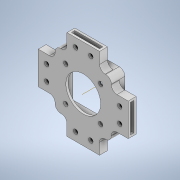
# Autodesk Inventor part: CSB_Motor_Mount_v1
Saved by Autodesk Inventor 2021 (Build 250183000, 183)
## iProperties
Created: 2023-12-30
Part Number: CSB_Motor_Mount_v1
Material: Generic
Document SubType Name: Modeling
Designer: brybr
Density: 1 g/cm^3
Appearance: Default
Author: brybr
Autodesk Inventor part; units mm, degrees
ref_plane "YZ Plane" through (0, 0, 0) normal (1, 0, 0) x (0, 1, 0)
ref_plane "XZ Plane" through (0, 0, 0) normal (0, 1, 0) x (-1, 0, 0)
ref_plane "XY Plane" through (0, 0, 0) normal (0, 0, 1) x (1, 0, 0)
sketch "Sketch1" plane through (0, 0, 0) normal (0, 0, 1) x (1, 0, 0)
  line L0 (-15.5, 15.5) -> (15.5, 15.5) construction
  line L1 (15.5, 15.5) -> (15.5, -15.5) construction
  line L2 (15.5, -15.5) -> (-15.5, -15.5) construction
  line L3 (-15.5, -15.5) -> (-15.5, 15.5) construction
  line L4 (-15.5, 15.5) -> (15.5, -15.5) construction
  line L5 (15.5, 15.5) -> (-15.5, -15.5) construction
  circle A0 centre (-15.5, 15.5) radius 2
  circle A1 centre (15.5, 15.5) radius 2
  circle A2 centre (-15.5, -15.5) radius 2
  circle A3 centre (15.5, -15.5) radius 2
  line L6 (-21.25, 21.25) -> (21.25, 21.25)
  line L7 (21.25, 21.25) -> (21.25, -21.25)
  line L8 (21.25, -21.25) -> (-21.25, -21.25)
  line L9 (-21.25, -21.25) -> (-21.25, 21.25)
  line L10 (-21.25, 21.25) -> (21.25, -21.25) construction
  line L11 (21.25, 21.25) -> (-21.25, -21.25) construction
  circle A4 centre (0, 0) radius 15.5
  line L12 (25, -25) -> (-25, -25)
  line L13 (-25, -25) -> (-25, 25)
  line L14 (-25, 25) -> (25, 25)
  line L15 (25, 25) -> (25, -25)
  line L16 (25, -25) -> (-25, 25) construction
  line L17 (-25, -25) -> (25, 25) construction
  dimension "d0" = 31
  dimension "d1" = 31
  dimension "d2" = 4
  dimension "d5" = 31
  dimension "d8" = 31
  dimension "d11" = 42.5
  dimension "d12" = 42.5
  dimension "d13" = 50
  dimension "d14" = 50
  constraints: 36 end point, 6 midpoint, 6 parallel, 5 centre point, 4 horizontal, 3 perpendicular, 2 coincident, 1 vertical, 6 other
  measures "d0" distance of L1.end L2.end
  measures "d1" distance of L0.end L1.end
  measures "d2" diameter of A0
  measures "d5" distance of A0.centre A1.centre
  measures "d8" distance of A0.centre A2.centre
  measures "d11" distance of L7.end L8.end
  measures "d12" distance of L6.end L7.end
  measures "d13" distance of L13.end L14.end
  measures "d14" distance of L12.end L13.end
extrude "Extrusion1" add sketch "Sketch1" along normal blind 2 contours L6 L7 L8 L9 | L12 L13 L14 L15
extrude "Extrusion2" add sketch "Sketch1" against normal blind 10 contours L12 L13 L14 L15
sketch "Sketch2" plane through (-25, -25, 2) normal (-1, 0, 0) x (0, 0, 1)
  line L0 (0, 0) -> (0, 50) construction
  line L1 (0, 0) -> (-2, 0) construction
  line L2 (-12, 0) -> (0, 0) construction
  line L3 (-2, 40.5) -> (-2, 9.5) construction
  line L4 (-2, 0) -> (-2, 25) construction
  line L5 (-2, 25) -> (-3.5, 25) construction
  line L6 (-5, 37.5) -> (-2, 37.5)
  line L7 (-2, 37.5) -> (-2, 12.5)
  line L8 (-2, 12.5) -> (-5, 12.5)
  line L9 (-5, 12.5) -> (-5, 37.5)
  line L10 (-5, 37.5) -> (-2, 12.5) construction
  line L11 (-2, 37.5) -> (-5, 12.5) construction
  line L12 (-7, 39.5) -> (0, 39.5)
  line L13 (0, 39.5) -> (0, 10.5)
  line L14 (0, 10.5) -> (-7, 10.5)
  line L15 (-7, 10.5) -> (-7, 39.5)
  dimension "d19" = 2
  dimension "d20" = 25
  dimension "d21" = 90
  dimension "d22" = 1.5
  dimension "d23" = 90
  dimension "d24" = 3
  dimension "d25" = 25
  dimension "d26" = 2
  dimension "d37" = 2
  constraints: 26 end point, 4 parallel, 3 perpendicular, 2 midpoint, 1 horizontal, 1 point on line, 3 other
  measures "d19" distance of L0.start L1.end
  measures "d20" distance of L1.end L4.end
  measures "d21" angle of L1 L4
  measures "d22" distance of L4.end L5.end
  measures "d23" angle of L5 L4
  measures "d24" distance of L7.end L8.end
  measures "d25" distance of L6.end L7.end
  measures "d26" distance between parallel lines of L9 L15
  measures "d37" distance between parallel lines of L7 L13
extrude "Extrusion3" add sketch "Sketch2" along normal blind 15
sketch "Sketch3" plane through (-25, -14.5, -5) normal (0, 0, -1) x (-1, 0, 0)
  line L0 (0, 0) -> (7.5, 0) construction
  line L1 (0, 0) -> (15, 0) construction
  line L2 (7.5, 14.5) -> (7.5, 21.25) construction
  line L3 (7.5, 21.25) -> (7.5, 7.75) construction
  circle A0 centre (7.5, 21.25) radius 2
  circle A1 centre (7.5, 7.75) radius 2
  line L4 (7.5, 0) -> (7.5, 7.75) construction
  line L5 (7.5, 21.25) -> (7.5, 29) construction
  line L6 (0, 29) -> (15, 29) construction
  point P0 (-25, 14.5)
  dimension "d30" = 4
  dimension "d31" = 4
  dimension "d38" = 13.5
  constraints: 10 end point, 2 centre point, 2 coincident, 2 collinear, 2 midpoint, 1 perpendicular, 1 vertical
  measures "d30" diameter of A0
  measures "d31" diameter of A1
  measures "d38" distance of L2.end L3.end
extrude "Extrusion4" cut sketch "Sketch3" against normal blind 15
pattern_circular "Circular Pattern1" count 4 over 360 about axis through (0, 0, -10) along (0, 0, 1) of "Extrusion3", "Extrusion4"
fillet "Fillet2" radius 5 12 edges at (25, 14.5, -1.5) (25, 25, -4) (14.5, 25, -1.5) (25, -14.5, -1.5) (14.5, -25, -1.5) (25, -25, -4) (-14.5, -25, -1.5) (-25, -25, -4) (-25, -14.5, -1.5) (-25, 14.5, -1.5) (-25, 25, -4) (-14.5, 25, -1.5)
body "Solid1"
